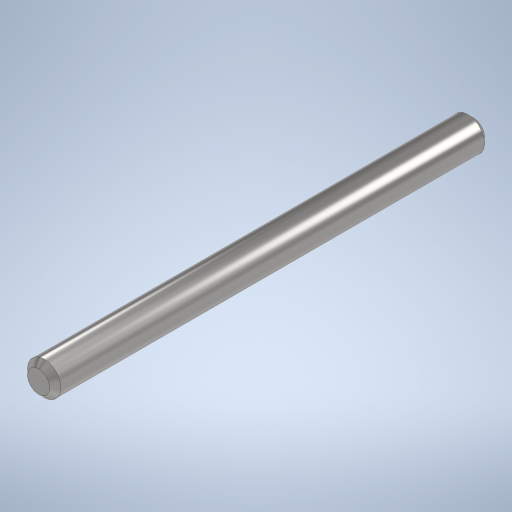
# Autodesk Inventor part: Main axel
Saved by Autodesk Inventor 2023 (Build 270158000, 158)
## iProperties
Created: 2022-05-02
Part Number: Main axel
Material: Stainless Steel
Document SubType Name: Modeling
Designer: Devin
Density: 8 g/cm^3
Appearance: Semi-Polished
Author: Devin
Autodesk Inventor part; units mm, degrees
ref_plane "YZ Plane" through (0, 0, 0) normal (1, 0, 0) x (0, 1, 0)
ref_plane "XZ Plane" through (0, 0, 0) normal (0, 1, 0) x (-1, 0, 0)
ref_plane "XY Plane" through (0, 0, 0) normal (0, 0, 1) x (1, 0, 0)
sketch "Sketch1" plane through (0, 0, 0) normal (0, 0, 1) x (1, 0, 0)
  circle A0 centre (0, 0) radius 0.762
  dimension "d0" = 1.524
  constraints: 1 centre point, 1 coincident
  measures "d0" diameter of A0
extrude "Extrusion1" add sketch "Sketch1" along normal blind 19.812
chamfer "Chamfer1" distance 0.254 distance2 0.254 1 edges at (-0.762, 0, 19.812) measured on face at (0.4109, -0.2521, 19.812)
chamfer "Chamfer2" distance 0.254 distance2 0.254 1 edges at (-0.762, 0, 0) measured on face at (0.7595, -0.0613, 13.0387)
body "Solid1"
